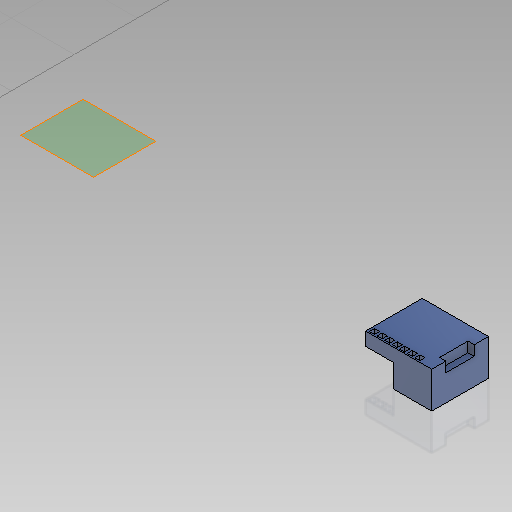
# Autodesk Inventor part: ЛЦМК0000002.00.00.00.00.04
Saved by Autodesk Inventor 2021.2 (Build 252289000, 289)
## iProperties
Created: 2025-10-23
Part Number: ЛЦМК0000002.00.00.00.00.04
Material: Типовые
Document SubType Name: Modeling
Designer: Захаров
Density: 1 g/cm^3
Appearance: С вкраплениями — сатинированная — синяя
Author: Захаров
Autodesk Inventor part; units mm, degrees
ref_plane "YZ Plane" through (0, 0, 0) normal (1, 0, 0) x (0, 1, 0)
ref_plane "XZ Plane" through (0, 0, 0) normal (0, 1, 0) x (-1, 0, 0)
ref_plane "XY Plane" through (0, 0, 0) normal (0, 0, 1) x (1, 0, 0)
ref_plane "РабПлоскость1" through (116.75, -2.8, -7.7) normal (0, -1, 0) x (1, 0, 0)
sketch "Эскиз1" plane through (116.75, -2.8, -7.7) normal (0, -1, 0) x (1, 0, 0)
  line L0 (104.15, 6.9) -> (102.55, 6.9) projected
  line L1 (102.55, 6.9) -> (102.55, 8.5) projected
  line L2 (102.55, 8.5) -> (104.15, 8.5) projected
  line L3 (104.15, 8.5) -> (104.15, 6.9) projected
  line L4 (99.35, 6.9) -> (97.75, 6.9) projected
  line L5 (97.75, 6.9) -> (97.75, 8.5) projected
  line L6 (97.75, 8.5) -> (99.35, 8.5) projected
  line L7 (99.35, 8.5) -> (99.35, 6.9) projected
  line L8 (108.95, 6.9) -> (107.35, 6.9) projected
  line L9 (107.35, 6.9) -> (107.35, 8.5) projected
  line L10 (107.35, 8.5) -> (108.95, 8.5) projected
  line L11 (108.95, 8.5) -> (108.95, 6.9) projected
  line L12 (106.55, 6.9) -> (104.95, 6.9) projected
  line L13 (104.95, 6.9) -> (104.95, 8.5) projected
  line L14 (104.95, 8.5) -> (106.55, 8.5) projected
  line L15 (106.55, 8.5) -> (106.55, 6.9) projected
  line L16 (111.35, 6.9) -> (109.75, 6.9) projected
  line L17 (109.75, 6.9) -> (109.75, 8.5) projected
  line L18 (109.75, 8.5) -> (111.35, 8.5) projected
  line L19 (111.35, 8.5) -> (111.35, 6.9) projected
  line L20 (101.75, 6.9) -> (100.15, 6.9) projected
  line L21 (100.15, 6.9) -> (100.15, 8.5) projected
  line L22 (100.15, 8.5) -> (101.75, 8.5) projected
  line L23 (101.75, 8.5) -> (101.75, 6.9) projected
  line L24 (113.75, 6.9) -> (112.15, 6.9) projected
  line L25 (112.15, 6.9) -> (112.15, 8.5) projected
  line L26 (112.15, 8.5) -> (113.75, 8.5) projected
  line L27 (113.75, 8.5) -> (113.75, 6.9) projected
  line L28 (116, 4.5) -> (118, 4.5) projected
  line L29 (118, 4.5) -> (118, 9) projected
  line L30 (118, 9) -> (97, 9) projected
  line L31 (97, 9) -> (97, -9) projected
  line L32 (97, -9) -> (118, -9) projected
  line L33 (118, -9) -> (118, -4.5) projected
  line L34 (118, -4.5) -> (116, -4.5) projected
  line L35 (116, -4.5) -> (116, 4.5) projected
  line L36 (102.55, -6.9) -> (104.15, -6.9) projected
  line L37 (104.15, -6.9) -> (104.15, -8.5) projected
  line L38 (104.15, -8.5) -> (102.55, -8.5) projected
  line L39 (102.55, -8.5) -> (102.55, -6.9) projected
  line L40 (97.75, -6.9) -> (99.35, -6.9) projected
  line L41 (99.35, -6.9) -> (99.35, -8.5) projected
  line L42 (99.35, -8.5) -> (97.75, -8.5) projected
  line L43 (97.75, -8.5) -> (97.75, -6.9) projected
  line L44 (107.35, -6.9) -> (108.95, -6.9) projected
  line L45 (108.95, -6.9) -> (108.95, -8.5) projected
  line L46 (108.95, -8.5) -> (107.35, -8.5) projected
  line L47 (107.35, -8.5) -> (107.35, -6.9) projected
  line L48 (104.95, -6.9) -> (106.55, -6.9) projected
  line L49 (106.55, -6.9) -> (106.55, -8.5) projected
  line L50 (106.55, -8.5) -> (104.95, -8.5) projected
  line L51 (104.95, -8.5) -> (104.95, -6.9) projected
  line L52 (109.75, -6.9) -> (111.35, -6.9) projected
  line L53 (111.35, -6.9) -> (111.35, -8.5) projected
  line L54 (111.35, -8.5) -> (109.75, -8.5) projected
  line L55 (109.75, -8.5) -> (109.75, -6.9) projected
  line L56 (100.15, -6.9) -> (101.75, -6.9) projected
  line L57 (101.75, -6.9) -> (101.75, -8.5) projected
  line L58 (101.75, -8.5) -> (100.15, -8.5) projected
  line L59 (100.15, -8.5) -> (100.15, -6.9) projected
  line L60 (112.15, -6.9) -> (113.75, -6.9) projected
  line L61 (113.75, -6.9) -> (113.75, -8.5) projected
  line L62 (113.75, -8.5) -> (112.15, -8.5) projected
  line L63 (112.15, -8.5) -> (112.15, -6.9) projected
  point P0 (-116.75, 7.7)
extrude "Выдавливание1" add sketch "Эскиз1" along normal blind 4.2 contours L35 L34 L33 L32 L31 L30 L29 L28 | L36 L37 L38 L39 | L40 L41 L42 L43 | L44 L45 L46 L47 | L48 L49 L50 L51 | L52 L53 L54 L55 | L56 L57 L58 L59 | L60 L61 L62 L63
sketch "Эскиз2" plane through (116.75, -7, -7.7) normal (0, -1, 0) x (1, 0, 0)
  line L0 (118, -9) -> (118, -4.5) projected
  line L1 (118, 9) -> (97, 9) projected
  line L2 (118, -9) -> (106, -9)
  line L3 (106, -9) -> (106, 9)
  line L4 (106, 9) -> (118, 9)
  line L5 (118, 9) -> (118, -9)
  point P0 (-116.75, 7.7)
  point P1 (118, -4.5)
  point P2 (118, 9)
  dimension "d2" = 12
  constraints: 8 end point, 2 parallel, 1 horizontal, 1 perpendicular, 1 point on line
  measures "d2" distance of L3.end L4.end
extrude "Выдавливание2" add sketch "Эскиз2" along normal blind 7.3
sketch "Эскиз3" plane through (116.75, -14.3, -7.7) normal (0, -1, 0) x (1, 0, 0)
  line L0 (102.55, 6.9) -> (104.15, 6.9) projected
  line L1 (104.15, 6.9) -> (104.15, 8.5) projected
  line L2 (104.15, 8.5) -> (102.55, 8.5) projected
  line L3 (102.55, 8.5) -> (102.55, 6.9) projected
  line L4 (97.75, 6.9) -> (99.35, 6.9) projected
  line L5 (99.35, 6.9) -> (99.35, 8.5) projected
  line L6 (99.35, 8.5) -> (97.75, 8.5) projected
  line L7 (97.75, 8.5) -> (97.75, 6.9) projected
  line L8 (107.35, 6.9) -> (108.95, 6.9) projected
  line L9 (108.95, 6.9) -> (108.95, 8.5) projected
  line L10 (108.95, 8.5) -> (107.35, 8.5) projected
  line L11 (107.35, 8.5) -> (107.35, 6.9) projected
  line L12 (104.95, 6.9) -> (106.55, 6.9) projected
  line L13 (106.55, 6.9) -> (106.55, 8.5) projected
  line L14 (106.55, 8.5) -> (104.95, 8.5) projected
  line L15 (104.95, 8.5) -> (104.95, 6.9) projected
  line L16 (109.75, 6.9) -> (111.35, 6.9) projected
  line L17 (111.35, 6.9) -> (111.35, 8.5) projected
  line L18 (111.35, 8.5) -> (109.75, 8.5) projected
  line L19 (109.75, 8.5) -> (109.75, 6.9) projected
  line L20 (100.15, 6.9) -> (101.75, 6.9) projected
  line L21 (101.75, 6.9) -> (101.75, 8.5) projected
  line L22 (101.75, 8.5) -> (100.15, 8.5) projected
  line L23 (100.15, 8.5) -> (100.15, 6.9) projected
  line L24 (112.15, 6.9) -> (113.75, 6.9) projected
  line L25 (113.75, 6.9) -> (113.75, 8.5) projected
  line L26 (113.75, 8.5) -> (112.15, 8.5) projected
  line L27 (112.15, 8.5) -> (112.15, 6.9) projected
  line L28 (118, 9) -> (97, 9) projected
  line L29 (118, -9) -> (118, 9) projected
  line L30 (97, -9) -> (118, -9) projected
  line L31 (97, 9) -> (97, -9) projected
  line L32 (104.15, -6.9) -> (102.55, -6.9) projected
  line L33 (102.55, -6.9) -> (102.55, -8.5) projected
  line L34 (102.55, -8.5) -> (104.15, -8.5) projected
  line L35 (104.15, -8.5) -> (104.15, -6.9) projected
  line L36 (99.35, -6.9) -> (97.75, -6.9) projected
  line L37 (97.75, -6.9) -> (97.75, -8.5) projected
  line L38 (97.75, -8.5) -> (99.35, -8.5) projected
  line L39 (99.35, -8.5) -> (99.35, -6.9) projected
  line L40 (108.95, -6.9) -> (107.35, -6.9) projected
  line L41 (107.35, -6.9) -> (107.35, -8.5) projected
  line L42 (107.35, -8.5) -> (108.95, -8.5) projected
  line L43 (108.95, -8.5) -> (108.95, -6.9) projected
  line L44 (106.55, -6.9) -> (104.95, -6.9) projected
  line L45 (104.95, -6.9) -> (104.95, -8.5) projected
  line L46 (104.95, -8.5) -> (106.55, -8.5) projected
  line L47 (106.55, -8.5) -> (106.55, -6.9) projected
  line L48 (111.35, -6.9) -> (109.75, -6.9) projected
  line L49 (109.75, -6.9) -> (109.75, -8.5) projected
  line L50 (109.75, -8.5) -> (111.35, -8.5) projected
  line L51 (111.35, -8.5) -> (111.35, -6.9) projected
  line L52 (101.75, -6.9) -> (100.15, -6.9) projected
  line L53 (100.15, -6.9) -> (100.15, -8.5) projected
  line L54 (100.15, -8.5) -> (101.75, -8.5) projected
  line L55 (101.75, -8.5) -> (101.75, -6.9) projected
  line L56 (113.75, -6.9) -> (112.15, -6.9) projected
  line L57 (112.15, -6.9) -> (112.15, -8.5) projected
  line L58 (112.15, -8.5) -> (113.75, -8.5) projected
  line L59 (113.75, -8.5) -> (113.75, -6.9) projected
  point P0 (-116.75, 7.7)
extrude "Выдавливание3" cut sketch "Эскиз3" against normal blind 7.3 contours L11 L10 L9 L8 | L15 L14 L13 L12 | L19 L18 L17 L16 | L27 L26 L25 L24
sketch "Эскиз4" plane through (116.75, -7, -7.7) normal (0, 1, 0) x (1, 0, 0)
  line L0 (116, -4.5) -> (118, -4.5) projected
  line L1 (118, 4.5) -> (118, -4.5) projected
  line L2 (118, 4.5) -> (116, 4.5) projected
  line L3 (116, 4.5) -> (116, -4.5) projected
  point P0 (-116.75, -7.7)
ref_plane "РабПлоскость2" through (10.25, -6, -12.2) normal (0, -1, 0) x (1, 0, 0)
extrude "Выдавливание4" add sketch "Эскиз4" along normal up to surface (1 mm away)
